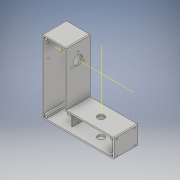
# Autodesk Inventor part: Main Lidar Body
Saved by Autodesk Inventor 2019 (Build 230136000, 136)
## iProperties
Created: 2018-05-20
Part Number: Main Lidar Body
Material: Generic
Document SubType Name: Modeling
Designer: samps
Density: 1 g/cm^3
Appearance: Default
Author: samps
Autodesk Inventor part; units mm, degrees
ref_plane "YZ Plane" through (0, 0, 0) normal (1, 0, 0) x (0, 1, 0)
ref_plane "XZ Plane" through (0, 0, 0) normal (0, 1, 0) x (-1, 0, 0)
ref_plane "XY Plane" through (0, 0, 0) normal (0, 0, 1) x (1, 0, 0)
sketch "Sketch2" plane through (0, 0, 0) normal (0, 0, 1) x (1, 0, 0)
  line L0 (0, 0) -> (0, 3.175)
  line L1 (0, 3.175) -> (50.8, 3.175)
  line L2 (50.8, 3.175) -> (53.975, 3.175)
  line L3 (53.975, 3.175) -> (53.975, -123.825)
  line L4 (53.975, -123.825) -> (108.712, -123.825)
  line L5 (108.712, -123.825) -> (163.449, -123.825)
  line L6 (163.449, -123.825) -> (166.624, -123.825)
  line L7 (166.624, -123.825) -> (166.624, -127)
  line L8 (166.624, -127) -> (166.624, -165.1)
  line L9 (166.624, -165.1) -> (166.624, -168.275)
  line L10 (166.624, -168.275) -> (163.449, -168.275)
  line L11 (163.449, -168.275) -> (0, -168.275)
  line L12 (0, -168.275) -> (-3.175, -168.275)
  line L13 (-3.175, -168.275) -> (-3.175, 0)
  line L14 (-3.175, 0) -> (-3.175, 3.175)
  line L15 (-3.175, 3.175) -> (0, 3.175)
  dimension "d6" = 3.175
  dimension "d13" = 3.175
  dimension "d16" = 3.175
  constraints: 32 end point, 7 point on line, 5 perpendicular, 2 vertical, 1 collinear, 1 horizontal
  measures "d6" distance of L0.start L0.end
  measures "d13" distance of L6.end L7.end
  measures "d16" distance of L9.end L10.end
extrude "Extrusion1" add sketch "Sketch2" along normal blind 55.5625
shell "Shell1" thickness 3.175 removed faces 1 at (15.875, -97.3667, 55.5625)
sketch "Sketch3" plane through (0, -165.1, 3.175) normal (0, 0, 1) x (1, 0, 0)
  line L0 (50.8, 38.1) -> (163.449, 38.1) projected
  line L1 (163.449, 0) -> (0, 0) projected
  line L2 (50.8, 38.1) -> (53.975, 38.1)
  line L3 (53.975, 38.1) -> (53.975, 0)
  line L4 (53.975, 0) -> (50.8, 0)
  line L5 (50.8, 0) -> (50.8, 38.1)
  point P0 (0, 165.1)
  dimension "d21" = 3.175
  constraints: 8 end point, 2 parallel, 1 horizontal, 1 perpendicular, 1 point on line
  measures "d21" distance of L3.end L4.end
extrude "Extrusion2" add sketch "Sketch3" along normal blind 38.1
sketch "Sketch4" plane through (0, 0, 3.175) normal (0, 0, 1) x (1, 0, 0)
  line L0 (0, 0) -> (50.8, 0) projected
  line L1 (0, 0) -> (6.8, 0)
  line L2 (6.8, 0) -> (6.8, -6.8)
  line L3 (6.8, -6.8) -> (0, -6.8)
  line L4 (0, -6.8) -> (0, 0)
  line L5 (50.8, 0) -> (44, 0)
  line L6 (44, 0) -> (44, -6.8)
  line L7 (44, -6.8) -> (50.8, -6.8)
  line L8 (50.8, -6.8) -> (50.8, 0)
  line L9 (0, -165.1) -> (0, 0) projected
  line L10 (0, -165.1) -> (6.8, -165.1)
  line L11 (6.8, -165.1) -> (6.8, -158.3)
  line L12 (6.8, -158.3) -> (0, -158.3)
  line L13 (0, -158.3) -> (0, -165.1)
  line L14 (50.8, -127) -> (163.449, -127) projected
  line L15 (53.9685, -127) -> (62.7685, -127)
  line L16 (62.7685, -127) -> (62.7685, -133.8)
  line L17 (62.7685, -133.8) -> (53.9685, -133.8)
  line L18 (53.9685, -133.8) -> (53.9685, -127)
  line L19 (163.449, -127) -> (163.449, -165.1) projected
  line L20 (163.449, -127) -> (156.649, -127)
  line L21 (156.649, -127) -> (156.649, -133.8)
  line L22 (156.649, -133.8) -> (163.449, -133.8)
  line L23 (163.449, -133.8) -> (163.449, -127)
  line L24 (163.449, -165.1) -> (156.649, -165.1)
  line L25 (156.649, -165.1) -> (156.649, -158.3)
  line L26 (156.649, -158.3) -> (163.449, -158.3)
  line L27 (163.449, -158.3) -> (163.449, -165.1)
  constraints: 48 end point, 12 parallel, 6 horizontal, 6 perpendicular, 1 point on line
extrude "Extrusion3" add sketch "Sketch4" along normal blind 50.8
sketch "Sketch5" plane through (0, 0, 53.975) normal (0, 0, 1) x (1, 0, 0)
  line L0 (0, -165.1) -> (0, 0) projected
  line L1 (0, 0) -> (2.15, 0)
  line L2 (2.15, 0) -> (2.15, -2.15)
  line L3 (2.15, -2.15) -> (0, -2.15)
  line L4 (0, -2.15) -> (0, 0)
  line L5 (50.8, 0) -> (50.8, -127) projected
  line L6 (50.8, 0) -> (48.65, 0)
  line L7 (48.65, 0) -> (48.65, -2.15)
  line L8 (48.65, -2.15) -> (50.8, -2.15)
  line L9 (50.8, -2.15) -> (50.8, 0)
  line L10 (163.449, -165.1) -> (0, -165.1) projected
  line L11 (0, -165.1) -> (2.15, -165.1)
  line L12 (2.15, -165.1) -> (2.15, -162.95)
  line L13 (2.15, -162.95) -> (0, -162.95)
  line L14 (0, -162.95) -> (0, -165.1)
  line L15 (53.9685, -127) -> (53.9685, -133.8) projected
  line L16 (53.9685, -127) -> (58.3685, -127)
  line L17 (62.7685, -133.8) -> (62.7685, -127) projected
  line L18 (58.3685, -127) -> (58.3685, -129.15)
  line L19 (50.8, -127) -> (163.449, -127) projected
  line L20 (163.449, -127) -> (161.299, -127)
  line L21 (161.299, -127) -> (161.299, -129.15)
  line L22 (161.299, -129.15) -> (163.449, -129.15)
  line L23 (163.449, -129.15) -> (163.449, -127)
  line L24 (163.449, -127) -> (163.449, -165.1) projected
  line L25 (163.449, -165.1) -> (161.299, -165.1)
  line L26 (161.299, -165.1) -> (161.299, -162.95)
  line L27 (161.299, -162.95) -> (163.449, -162.95)
  line L28 (163.449, -162.95) -> (163.449, -165.1)
  constraints: 44 end point, 10 parallel, 7 perpendicular, 5 horizontal, 1 point on line
hole "Hole1" at (2.15, -2.15, 53.975) at (48.65, -2.15, 53.975) at (2.15, -162.95, 53.975) at (58.3685, -129.15, 53.975) at (161.299, -129.15, 53.975) at (161.299, -162.95, 53.975) direction (0, 0, -1) diameter 3.5 depth 3.5
fillet "Fillet1" radius 2 5 edges at (53.975, 3.175, 27.7812) (166.624, -123.825, 27.7812) (166.624, -168.275, 27.7812) (-3.175, -168.275, 27.7812) (-3.175, 3.175, 27.7812)
fillet "Fillet2" radius 2 7 edges at (6.8, -158.3, 28.575) (6.8, -6.8, 28.575) (44, -6.8, 28.575) (62.7685, -133.8, 28.575) (53.9685, -133.8, 47.625) (156.649, -158.3, 28.575) (156.649, -133.8, 28.575)
sketch "Sketch6" plane through (53.975, -123.825, 55.5625) normal (1, 0, 0) x (0, 0, -1)
  line L0 (52.3875, 123.825) -> (1.5875, 123.825) projected
  line L1 (52.3875, 123.825) -> (52.3875, 88.825)
  line L2 (52.3875, -34.475) -> (52.3875, 117.025) projected
  line L3 (52.3875, 88.825) -> (26.9875, 88.825)
  line L4 (0, 123.825) -> (0, -3.175) projected
  point P0 (55.5625, 123.825)
  dimension "d58" = 35
  dimension "d59" = 25.4
  constraints: 4 end point, 1 perpendicular, 1 point on line
  measures "d58" distance of L0.start L1.end
  measures "d59" distance of L1.end L3.end
hole "Hole2" at (53.975, -35, 28.575) direction (-1, 0, 0) diameter 22 depth 3.175
sketch "Sketch7" plane through (53.975, -123.825, 55.5625) normal (0, 1, 0) x (1, 0, 0)
  line L0 (0, 52.3875) -> (0, 14.2875) projected
  line L1 (0, 52.3875) -> (54.737, 52.3875)
  line L2 (102.674, 52.3875) -> (0, 52.3875) projected
  line L3 (54.737, 52.3875) -> (54.737, 26.9875)
  point P0 (-53.975, 55.5625)
  dimension "d67" = 54.737
  dimension "d68" = 25.4
  constraints: 4 end point, 1 perpendicular, 1 point on line
  measures "d67" distance of L0.start L1.end
  measures "d68" distance of L1.end L3.end
hole "Hole3" at (108.712, -123.825, 28.575) direction (0, -1, 0) diameter 15.5 end through all
sketch "Sketch8" plane through (53.975, -123.825, 55.5625) normal (1, 0, 0) x (0, 0, -1)
  circle A0 centre (26.9875, 88.825) radius 11 projected
  line L0 (26.9875, 88.825) -> (26.9875, 106.275)
  line L1 (26.9875, 88.825) -> (42.0996, 80.1)
  line L2 (26.9875, 88.825) -> (44.4375, 88.825) construction
  line L3 (26.9875, 88.825) -> (11.8754, 80.1)
  line L4 (26.9875, 88.825) -> (44.4375, 88.825) construction
  point P0 (55.5625, 123.825)
  dimension "d76" = 17.45
  dimension "d77" = 17.45
  dimension "d78" = 30
  dimension "d79" = 17.45
  dimension "d80" = 150
  constraints: 10 end point, 2 equal length, 2 horizontal, 1 vertical
  measures "d76" distance of L0.start L0.end
  measures "d77" distance of L0.start L1.end
  measures "d78" angle of L1 L2
  measures "d79" distance of L0.start L3.end
  measures "d80" angle of L3 L4
hole "Hole4" at (53.975, -17.55, 28.575) at (53.975, -43.725, 13.4629) at (53.975, -43.725, 43.6871) direction (-1, 0, 0) diameter 3.5 depth 3.175
sketch "Sketch9" plane through (-3.175, -166.275, 0) normal (-1, 0, 0) x (0, 0, 1)
  circle A0 centre (28.575, 131.275) radius 11 projected
  line L0 (28.575, 146.775) -> (13.075, 146.775)
  line L1 (13.075, 146.775) -> (44.075, 146.775)
  line L2 (44.075, 146.775) -> (44.075, 115.775)
  line L3 (44.075, 115.775) -> (13.075, 115.775)
  line L4 (13.075, 115.775) -> (13.075, 146.775)
  point P0 (0, 166.275)
  dimension "d90" = 31
  dimension "d91" = 31
  constraints: 10 end point, 2 parallel, 1 coincident, 1 horizontal, 1 perpendicular
  measures "d90" distance of L2.end L3.end
  measures "d91" distance of L1.end L2.end
hole "Hole5" at (-3.175, -50.5, 13.075) at (-3.175, -19.5, 13.075) at (-3.175, -19.5, 44.075) at (-3.175, -50.5, 44.075) direction (1, 0, 0) diameter 3 depth 3.175
sketch "Sketch10" plane through (50.8, -127, 55.5625) normal (-1, 0, 0) x (0, 0, 1)
  line L0 (-14.2875, -38.1) -> (-52.3875, -38.1) projected
  line L1 (-52.3875, -38.1) -> (-38.2875, -38.1)
  line L2 (-38.2875, -38.1) -> (-38.2875, -24)
  line L3 (-38.2875, -24) -> (-38.2875, -12.5)
  line L4 (-38.2875, -12.5) -> (-49.7875, -12.5)
  line L5 (-49.7875, -12.5) -> (-26.7875, -12.5)
  line L6 (-26.7875, -12.5) -> (-26.7875, -35.5)
  line L7 (-26.7875, -35.5) -> (-49.7875, -35.5)
  line L8 (-49.7875, -35.5) -> (-49.7875, -12.5)
  point P0 (-55.5625, 127)
  dimension "d99" = 14.1
  dimension "d100" = 14.1
  dimension "d101" = 11.5
  dimension "d102" = 11.5
  dimension "d103" = 23
  dimension "d104" = 23
  constraints: 16 end point, 2 horizontal, 2 parallel, 2 perpendicular, 2 point on line
  measures "d99" distance of L0.end L1.end
  measures "d100" distance of L1.end L2.end
  measures "d101" distance of L2.end L3.end
  measures "d102" distance of L3.end L4.end
  measures "d103" distance of L6.end L7.end
  measures "d104" distance of L5.end L6.end
hole "Hole6" at (50.8, -139.5, 5.775) at (50.8, -139.5, 28.775) at (50.8, -162.5, 28.775) at (50.8, -162.5, 5.775) direction (1, 0, 0) diameter 2.5 depth 3.175
sketch "Sketch11" plane through (166.624, -166.275, 0) normal (1, 0, 0) x (0, 0, -1)
  line L0 (-53.975, 39.275) -> (-53.975, 34.475) projected
  line L1 (-53.975, 39.275) -> (-49.575, 39.275)
  line L2 (-3.175, 39.275) -> (-53.975, 39.275) projected
  line L3 (-49.575, 39.275) -> (-49.575, 37.125)
  line L4 (-50.475, 38.875) -> (-50.475, 35.375) projected
  line L5 (-3.175, 34.475) -> (-3.175, 39.275) projected
  line L6 (-3.175, 39.275) -> (-7.575, 39.275)
  line L7 (-7.575, 39.275) -> (-7.575, 37.125)
  line L8 (-53.975, 1.175) -> (-3.175, 1.175) projected
  line L9 (-53.975, 1.175) -> (-49.575, 1.175)
  line L10 (-49.575, 1.175) -> (-49.575, 3.325)
  line L11 (-3.175, 1.175) -> (-3.175, 5.975) projected
  line L12 (-3.175, 1.175) -> (-7.575, 1.175)
  line L13 (-7.575, 1.175) -> (-7.575, 3.325)
  point P0 (0, 166.275)
  dimension "d112" = 4.4
  dimension "d113" = 2.15
  dimension "d114" = 90
  dimension "d115" = 4.4
  dimension "d116" = 2.15
  dimension "d117" = 4.4
  dimension "d118" = 2.15
  dimension "d119" = 4.4
  dimension "d120" = 2.15
  constraints: 16 end point, 4 point on line, 3 perpendicular, 1 parallel
  measures "d112" distance of L0.start L1.end
  measures "d113" distance of L1.end L3.end
  measures "d114" angle of L1 L3
  measures "d115" distance of L2.start L6.end
  measures "d116" distance of L6.end L7.end
  measures "d117" distance of L8.start L9.end
  measures "d118" distance of L9.end L10.end
  measures "d119" distance of L8.end L12.end
  measures "d120" distance of L12.end L13.end
hole "Hole7" at (166.624, -129.15, 49.575) at (166.624, -129.15, 7.575) at (166.624, -162.95, 49.575) at (166.624, -162.95, 7.575) direction (-1, 0, 0) diameter 3.5 depth 3.175
body "Solid1"
